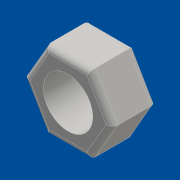
# Autodesk Inventor part: Tuerca
Saved by Autodesk Inventor 2016 (Build 200138000, 138)
## iProperties
Created: 2017-05-13
Part Number: Tuerca
Material: Generic
Document SubType Name: Modeling
Designer: Gian
Density: 1 g/cm^3
Appearance: Default
Author: Gian
Autodesk Inventor part; units mm, degrees
ref_plane "YZ Plane" through (0, 0, 0) normal (1, 0, 0) x (0, 1, 0)
ref_plane "XZ Plane" through (0, 0, 0) normal (0, 1, 0) x (-1, 0, 0)
ref_plane "XY Plane" through (0, 0, 0) normal (0, 0, 1) x (1, 0, 0)
sketch "Sketch1" plane through (0, 0, 0) normal (0, 1, 0) x (-1, 0, 0)
  line L0 (-0.4861, -7.0529) -> (-8.569, -7.0529)
  line L1 (-8.569, -7.0529) -> (-12.6104, -0.0529)
  line L2 (-12.6104, -0.0529) -> (-8.569, 6.9471)
  line L3 (-8.569, 6.9471) -> (-0.4861, 6.9471)
  line L4 (-0.4861, 6.9471) -> (3.5554, -0.0529)
  line L5 (3.5554, -0.0529) -> (-0.4861, -7.0529)
  circle A0 centre (-4.5275, -0.0529) radius 4.5
  dimension "d0" = 14
  dimension "d1" = 9
  constraints: 12 end point, 1 centre point, 1 coincident, 1 horizontal, 13 other
  measures "d0" distance between parallel lines of L0 L3
  measures "d1" diameter of A0
extrude "Extrusion1" add sketch "Sketch1" along normal blind 8
fillet "Fillet1" radius 1 12 edges at (4.5275, 8, 6.9471) (10.5897, 8, 3.4471) (10.5897, 8, -3.5529) (4.5275, 8, -7.0529) (-1.5346, 8, -3.5529) (-1.5346, 8, 3.4471) (4.5275, 0, 6.9471) (10.5897, 0, 3.4471) (10.5897, 0, -3.5529) (4.5275, 0, -7.0529) (-1.5346, 0, -3.5529) (-1.5346, 0, 3.4471)
body "Solid1"
